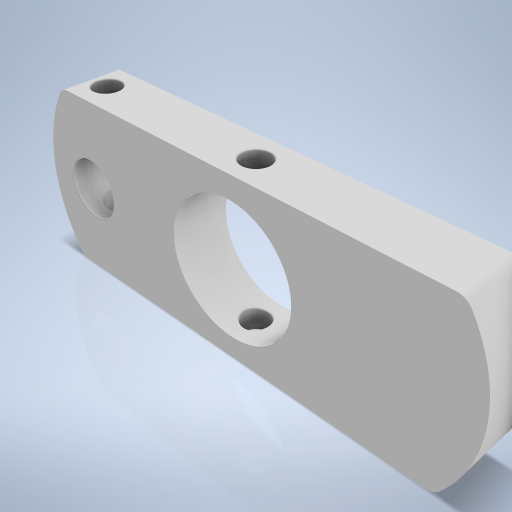
# Autodesk Inventor part: wheel_support
Saved by Autodesk Inventor 2024.2 (Build 282272000, 272)
## iProperties
Created: 2024-05-05
Part Number: wheel_support
Material: Generisch
Document SubType Name: Modeling
Designer: Fabri
Density: 1 g/cm^3
Appearance: Vorgabe
Author: Fabri
Autodesk Inventor part; units mm, degrees
ref_plane "YZ Plane" through (0, 0, 0) normal (1, 0, 0) x (0, 1, 0)
ref_plane "XZ Plane" through (0, 0, 0) normal (0, 1, 0) x (-1, 0, 0)
ref_plane "XY Plane" through (0, 0, 0) normal (0, 0, 1) x (1, 0, 0)
sketch "Skizze1" plane through (0, 0, 0) normal (0, 1, 0) x (-1, 0, 0)
  line L0 (10.0667, 24) -> (117.9333, 24)
  line L1 (117.9333, -24) -> (10.0667, -24)
  line L2 (0, 0) -> (128, 0) construction
  arc A0 (6.7408, 22.2222) -> (6.7408, -22.2222) centre (40, 0) ccw
  arc A1 (121.2592, -22.2222) -> (121.2592, 22.2222) centre (88, 0) ccw
  arc A2 (121.2592, 22.2222) -> (117.9333, 24) centre (117.9333, 20) ccw
  arc A3 (117.9333, -24) -> (121.2592, -22.2222) centre (117.9333, -20) ccw
  arc A4 (6.7408, -22.2222) -> (10.0667, -24) centre (10.0667, -20) ccw
  arc A5 (10.0667, 24) -> (6.7408, 22.2222) centre (10.0667, 20) ccw
  point P0 (120, -24)
  point P1 (120, -24)
  point P2 (120, -24)
  point P3 (120, 24)
  point P4 (120, 24)
  point P5 (120, 24)
  point P6 (8, -24)
  point P7 (8, -24)
  point P8 (8, -24)
  point P9 (8, 24)
  point P10 (8, 24)
  point P11 (8, 24)
  point P12 (128, 0)
  dimension "d1" = 0
  dimension "d3" = 0
  dimension "d2" = 48
  dimension "d24" = 128
  dimension "d25" = 4
  dimension "d26" = 40
  dimension "d27" = 40
  constraints: 18 point on circle, 8 tangent, 6 centre point, 6 end point, 5 horizontal, 4 point on line, 3 equal radius, 2 coincident, 2 symmetric about line, 16 other
  measures "d2" distance between parallel lines of L1 L0
  measures "d24" distance of L2.start point (128, 0)
  measures "d25" radius of A2
  measures "d26" radius of A1
  measures "d27" radius of A0
extrude "Extrusion1" add sketch "Skizze1" along normal blind 16
sketch "Skizze2" plane through (0, 0, 0) normal (0, 1, 0) x (1, 0, 0)
  line L0 (-117.9333, -24) -> (-10.0667, -24) projected
  arc A0 (-121.2592, 22.2222) -> (-121.2592, -22.2222) centre (-88, 0) ccw projected
  point P0 (0, 0)
  point P1 (-64, 0)
  point P2 (2, 0)
  point P3 (-112, 0)
  point P4 (2, 0)
  point P5 (-128, 0)
  point P6 (-64, -24)
  dimension "d29" = 48
  constraints: 4 horizontal alignment, 1 midpoint, 1 point on circle, 1 vertical alignment
  measures "d29" distance of point (-64, 0) point (-112, 0)
hole "Bohrung1" at (-64, 0, 0) direction (0, 1, 0) diameter 36 depth 16
hole "Bohrung2" at (-112, 0, 0) direction (0, 1, 0) diameter 16 depth 16
sketch "Skizze3" plane through (-10.0667, 0, -24) normal (0, 0, -1) x (-1, 0, 0)
  line L0 (0, 0) -> (0, 16) projected
  line L1 (111.1924, 0) -> (111.1924, 16) projected
  line L2 (0, 0) -> (107.8665, 0) projected
  point P0 (-10.0667, 0)
  point P1 (103.1924, 8)
  point P2 (0, 8)
  point P3 (53.9333, 8)
  point P4 (53.9333, 0)
  dimension "d37" = 8
  constraints: 2 horizontal alignment, 2 midpoint, 1 vertical alignment
  measures "d37" distance from line of point (103.192, 8) L1
hole "Bohrung3" at (-113.2592, 8, -24) direction (0, 0, 1) diameter 8 end through all
hole "Bohrung4" at (-64, 8, -24) direction (0, 0, 1) diameter 8 end through all
